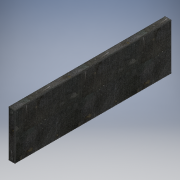
# Autodesk Inventor part: 内层侧板
Saved by Autodesk Inventor 2017 (Build 210142000, 142)
## iProperties
Part Number: 内层侧板
Material: 常规
Document SubType Name: Modeling
Designer: PANDA
Density: 1 g/cm^3
Appearance: 板
Author: PANDA
Autodesk Inventor part; units mm, degrees
ref_plane "YZ Plane" through (0, 0, 0) normal (1, 0, 0) x (0, 1, 0)
ref_plane "XZ Plane" through (0, 0, 0) normal (0, 1, 0) x (-1, 0, 0)
ref_plane "XY Plane" through (0, 0, 0) normal (0, 0, 1) x (1, 0, 0)
sketch "草图1" plane through (0, 0, 0) normal (0, 0, 1) x (1, 0, 0)
  point P0 (0, 0)
sketch "草图2" plane through (0, 0, 0) normal (1, 0, 0) x (0, 1, 0)
  line L0 (200, 70) -> (-200, 70)
  line L1 (-200, 70) -> (-200, -70)
  line L2 (-200, -70) -> (200, -70)
  line L3 (200, -70) -> (200, 70)
  point P0 (0, 0)
  dimension "d0" = 400
  dimension "d1" = 140
  constraints: 8 end point, 2 parallel, 1 horizontal, 1 perpendicular
  measures "d0" distance of L2.end L1.end
  measures "d1" distance of L1.end L0.end
extrude "拉伸1" add sketch "草图2" along normal blind 20
sketch "草图3" plane through (0, -200, -70) normal (0, -1, 0) x (1, 0, 0)
  circle A0 centre (10, 10) radius 2
  point P0 (0, 70)
  dimension "d4" = 4
  constraints: 1 centre point
  measures "d4" diameter of A0
extrude "拉伸2" cut sketch "草图3" against normal blind 40
sketch "草图4" plane through (0, -200, -70) normal (0, -1, 0) x (1, 0, 0)
  circle A0 centre (10, 130) radius 2
  point P0 (0, 70)
  dimension "d7" = 4
  constraints: 1 centre point
  measures "d7" diameter of A0
extrude "拉伸3" cut sketch "草图4" against normal blind 40
sketch "草图5" plane through (0, 200, 70) normal (0, 1, 0) x (1, 0, 0)
  line L0 (20, 0) -> (20, 140) projected
  line L1 (20, 140) -> (0, 140)
  line L2 (0, 140) -> (0, 0)
  line L3 (0, 0) -> (20, 0)
  line L4 (20, 0) -> (20, 140)
  point P0 (0, 70)
  constraints: 8 end point, 2 parallel, 1 horizontal, 1 perpendicular
extrude "拉伸4" add sketch "草图5" along normal blind 50
sketch "草图6" plane through (0, 250, 70) normal (0, 1, 0) x (1, 0, 0)
  line L0 (0, 0) -> (20, 0) projected
  line L1 (20, 140) -> (0, 140) projected
  line L2 (20, 0) -> (0, 0)
  line L3 (0, 0) -> (0, 140)
  line L4 (0, 140) -> (20, 140)
  line L5 (20, 140) -> (20, 0)
  point P0 (0, 70)
  constraints: 8 end point, 2 parallel, 1 horizontal, 1 perpendicular
extrude "拉伸5" add sketch "草图6" along normal blind 20
fillet "圆角1" radius 2 2 edges at (8, -160, 60) (8, -160, -60)
fillet "圆角1" radius 2 14 edges at (10, 270, 70) (0, 35, 70) (10, -200, 70) (20, 35, 70) (20, 270, 0) (20, -200, 0) (20, 35, -70) (0, 270, 0) (0, 35, -70) (0, -200, 0) (10, 270, -70) (10, -200, -70) (8, -200, 60) (8, -200, -60)
